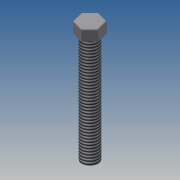
# Autodesk Inventor part: lagBolt_38
Saved by Autodesk Inventor 2014 SP1 (Build 180222100, 222)
## iProperties
Created: 2014-08-29
Part Number: lagBolt_38
Material: Generic
Document SubType Name: Modeling
Designer: Dave
Density: 1 g/cm^3
Appearance: Default
Author: Dave
Autodesk Inventor part; units mm, degrees
ref_plane "YZ Plane" through (0, 0, 0) normal (1, 0, 0) x (0, 1, 0)
ref_plane "XZ Plane" through (0, 0, 0) normal (0, 1, 0) x (-1, 0, 0)
ref_plane "XY Plane" through (0, 0, 0) normal (0, 0, 1) x (1, 0, 0)
sketch "Sketch1" plane through (0, 0, 0) normal (0, 1, 0) x (-1, 0, 0)
  line L0 (-1.7583, 6.772) -> (4.9856, 4.9088)
  line L1 (4.9856, 4.9088) -> (6.7439, -1.8632)
  line L2 (6.7439, -1.8632) -> (1.7583, -6.772)
  line L3 (1.7583, -6.772) -> (-4.9856, -4.9088)
  line L4 (-4.9856, -4.9088) -> (-6.7439, 1.8632)
  line L5 (-6.7439, 1.8632) -> (-1.7583, 6.772)
  point P0 (0, 0)
  point P1 (0, 0)
  constraints: 12 end point, 1 coincident, 13 other
extrude "Extrusion1" add sketch "Sketch1" along normal blind 6.35
fillet "Fillet1" radius 0.762 6 edges at (4.2511, 6.35, 4.3176) (5.8647, 6.35, -1.5228) (1.6136, 6.35, -5.8404) (-4.2511, 6.35, -4.3176) (-5.8647, 6.35, 1.5228) (-1.6136, 6.35, 5.8404)
sketch "Sketch2" plane through (0, 0, 0) normal (0, -1, 0) x (1, 0, 0)
  circle A0 centre (0, 0) radius 4.6482
  dimension "d3" = 9.2964
  constraints: 1 centre point, 1 coincident
  measures "d3" diameter of A0
extrude "Extrusion2" add sketch "Sketch2" along normal blind 63.5
thread "Thread1" size "3/8-16 UNC" class "2A" standard "ANSI Unified Screw Threads" full length
body "Solid1"
